Autodesk Inventor part; units mm, degrees
(part 4 of 4)
  spline S791 degree 2 poles (-83.876, -10.5733) (-84.1775, -10.5733) (-84.5737, -10.1697) (-84.5737, -9.8634) knots 0 0 0 1 2 2 2
  spline S792 degree 2 poles (-84.5737, -9.8634) (-84.5737, -9.613) (-84.372, -9.3018) (-84.1823, -9.2118) knots 0 0 0 1 2 2 2
  spline S793 degree 2 poles (-84.1823, -9.2118) (-83.9903, -9.1195) (-83.4579, -9.0465) (-83.1515, -9.0271) knots 0 0 0 1 2 2 2
  line L809 (-83.1515, -9.0271) -> (-83.1515, -9.0149)
  spline S794 degree 2 poles (-83.1515, -9.0149) (-83.1515, -8.8277) (-83.4287, -8.6843) (-83.7058, -8.6843) knots 0 0 0 1 2 2 2
  spline S795 degree 2 poles (-83.7058, -8.6843) (-83.8298, -8.6843) (-84.1653, -8.7742) (-84.3233, -8.8447) knots 0 0 0 1 2 2 2
  line L810 (-84.3233, -8.8447) -> (-84.3841, -8.8447)
  line L811 (-84.3841, -8.8447) -> (-84.3841, -8.2977)
  spline S796 degree 2 poles (-84.3841, -8.2977) (-84.2796, -8.2686) (-83.8128, -8.1859) (-83.5746, -8.1859) knots 0 0 0 1 2 2 2
  spline S797 degree 2 poles (-83.5746, -8.1859) (-82.9911, -8.1859) (-82.4562, -8.5749) (-82.4562, -8.9736) knots 0 0 0 1 2 2 2
  line L812 (-82.4562, -8.9736) -> (-82.4562, -10.5125)
  line L813 (-82.4562, -10.5125) -> (-83.1564, -10.5125)
  line L814 (-83.1564, -10.5125) -> (-83.1564, -10.2718)
  line L815 (-83.1564, -9.9217) -> (-83.1564, -9.4525)
  spline S798 degree 2 poles (-83.1564, -9.4525) (-83.3363, -9.4695) (-83.5575, -9.4963) (-83.6645, -9.5352) knots 0 0 0 1 2 2 2
  spline S799 degree 2 poles (-83.6645, -9.5352) (-83.7593, -9.5668) (-83.8614, -9.6981) (-83.8614, -9.805) knots 0 0 0 1 2 2 2
  spline S800 degree 2 poles (-83.8614, -9.805) (-83.8614, -9.9631) (-83.6888, -10.0822) (-83.5211, -10.0822) knots 0 0 0 1 2 2 2
  spline S801 degree 2 poles (-83.5211, -10.0822) (-83.4287, -10.0822) (-83.2342, -9.9971) (-83.1564, -9.9217) knots 0 0 0 1 2 2 2
  line L816 (-79.816, -10.5125) -> (-80.5259, -10.5125)
  line L817 (-80.5259, -10.5125) -> (-80.5259, -9.3917)
  spline S802 degree 2 poles (-80.5259, -9.3917) (-80.5259, -9.2532) (-80.5478, -8.9809) (-80.577, -8.9177) knots 0 0 0 1 2 2 2
  spline S803 degree 2 poles (-80.577, -8.9177) (-80.6135, -8.8399) (-80.7496, -8.7742) (-80.8663, -8.7742) knots 0 0 0 1 2 2 2
  spline S804 degree 2 poles (-80.8663, -8.7742) (-80.9514, -8.7742) (-81.1288, -8.8399) (-81.2285, -8.9104) knots 0 0 0 1 2 2 2
  line L818 (-81.2285, -8.9104) -> (-81.2285, -10.5125)
  line L819 (-81.2285, -10.5125) -> (-81.9335, -10.5125)
  line L820 (-81.9335, -10.5125) -> (-81.9335, -8.2491)
  line L821 (-81.9335, -8.2491) -> (-81.2285, -8.2491)
  line L822 (-81.2285, -8.2491) -> (-81.2285, -8.4995)
  spline S805 degree 2 poles (-81.2285, -8.4995) (-81.0559, -8.3537) (-80.7277, -8.1883) (-80.5284, -8.1883) knots 0 0 0 1 2 2 2
  spline S806 degree 2 poles (-80.5284, -8.1883) (-80.1831, -8.1883) (-79.816, -8.6259) (-79.816, -9.0392) knots 0 0 0 1 2 2 2
  line L823 (-79.816, -9.0392) -> (-79.816, -10.5125)
  line L824 (-78.5883, -10.5125) -> (-79.2934, -10.5125)
  line L825 (-79.2934, -10.5125) -> (-79.2934, -8.2491)
  line L826 (-79.2934, -8.2491) -> (-78.5883, -8.2491)
  line L827 (-78.5883, -8.2491) -> (-78.5883, -10.5125)
  line L828 (-78.5664, -7.9258) -> (-79.3128, -7.9258)
  line L829 (-79.3128, -7.9258) -> (-79.3128, -7.3763)
  line L830 (-79.3128, -7.3763) -> (-78.5664, -7.3763)
  line L831 (-78.5664, -7.3763) -> (-78.5664, -7.9258)
  spline S807 degree 2 poles (-76.94, -10.5733) (-77.2196, -10.5733) (-77.684, -10.4323) (-77.8566, -10.2864) knots 0 0 0 1 2 2 2
  spline S808 degree 2 poles (-77.8566, -10.2864) (-78.0243, -10.1381) (-78.2139, -9.6932) (-78.2139, -9.3917) knots 0 0 0 1 2 2 2
  spline S809 degree 2 poles (-78.2139, -9.3917) (-78.2139, -9.066) (-78.0097, -8.6114) (-77.8323, -8.4655) knots 0 0 0 1 2 2 2
  spline S810 degree 2 poles (-77.8323, -8.4655) (-77.6645, -8.3245) (-77.2075, -8.1883) (-76.9595, -8.1883) knots 0 0 0 1 2 2 2
  spline S811 degree 2 poles (-76.9595, -8.1883) (-76.7723, -8.1883) (-76.3979, -8.2759) (-76.2083, -8.3707) knots 0 0 0 1 2 2 2
  line L832 (-76.2083, -8.3707) -> (-76.2083, -8.9736)
  line L833 (-76.2083, -8.9736) -> (-76.2982, -8.9736)
  spline S812 degree 2 poles (-76.2982, -8.9736) (-76.342, -8.9323) (-76.4635, -8.835) (-76.5365, -8.7961) knots 0 0 0 1 2 2 2
  spline S813 degree 2 poles (-76.5365, -8.7961) (-76.6143, -8.7524) (-76.8063, -8.694) (-76.9254, -8.694) knots 0 0 0 1 2 2 2
  spline S814 degree 2 poles (-76.9254, -8.694) (-77.1953, -8.694) (-77.4919, -9.0708) (-77.4919, -9.3917) knots 0 0 0 1 2 2 2
  spline S815 degree 2 poles (-77.4919, -9.3917) (-77.4919, -9.7321) (-77.1759, -10.0676) (-76.9133, -10.0676) knots 0 0 0 1 2 2 2
  spline S816 degree 2 poles (-76.9133, -10.0676) (-76.7796, -10.0676) (-76.5802, -10.0068) (-76.5073, -9.9631) knots 0 0 0 1 2 2 2
  spline S817 degree 2 poles (-76.5073, -9.9631) (-76.4368, -9.9217) (-76.3347, -9.8293) (-76.2982, -9.7929) knots 0 0 0 1 2 2 2
  line L834 (-76.2982, -9.7929) -> (-76.2083, -9.7929)
  line L835 (-76.2083, -9.7929) -> (-76.2083, -10.3982)
  spline S818 degree 2 poles (-76.2083, -10.3982) (-76.269, -10.425) (-76.4271, -10.493) (-76.5097, -10.5149) knots 0 0 0 1 2 2 2
  spline S819 degree 2 poles (-76.5097, -10.5149) (-76.6118, -10.5441) (-76.7917, -10.5733) (-76.94, -10.5733) knots 0 0 0 1 2 2 2
  spline S820 degree 2 poles (-74.6256, -10.2718) (-74.6985, -10.3326) (-74.8128, -10.4298) (-74.91, -10.4785) knots 0 0 0 1 2 2 2
  spline S821 degree 2 poles (-74.91, -10.4785) (-75.0049, -10.5246) (-75.1848, -10.5733) (-75.3452, -10.5733) knots 0 0 0 1 2 2 2
  spline S822 degree 2 poles (-75.3452, -10.5733) (-75.6467, -10.5733) (-76.0429, -10.1697) (-76.0429, -9.8634) knots 0 0 0 1 2 2 2
  spline S823 degree 2 poles (-76.0429, -9.8634) (-76.0429, -9.613) (-75.8412, -9.3018) (-75.6515, -9.2118) knots 0 0 0 1 2 2 2
  spline S824 degree 2 poles (-75.6515, -9.2118) (-75.4595, -9.1195) (-74.9271, -9.0465) (-74.6207, -9.0271) knots 0 0 0 1 2 2 2
  line L836 (-74.6207, -9.0271) -> (-74.6207, -9.0149)
  spline S825 degree 2 poles (-74.6207, -9.0149) (-74.6207, -8.8277) (-74.8979, -8.6843) (-75.175, -8.6843) knots 0 0 0 1 2 2 2
  spline S826 degree 2 poles (-75.175, -8.6843) (-75.299, -8.6843) (-75.6345, -8.7742) (-75.7925, -8.8447) knots 0 0 0 1 2 2 2
  line L837 (-75.7925, -8.8447) -> (-75.8533, -8.8447)
  line L838 (-75.8533, -8.8447) -> (-75.8533, -8.2977)
  spline S827 degree 2 poles (-75.8533, -8.2977) (-75.7488, -8.2686) (-75.282, -8.1859) (-75.0438, -8.1859) knots 0 0 0 1 2 2 2
  spline S828 degree 2 poles (-75.0438, -8.1859) (-74.4603, -8.1859) (-73.9254, -8.5749) (-73.9254, -8.9736) knots 0 0 0 1 2 2 2
  line L839 (-73.9254, -8.9736) -> (-73.9254, -10.5125)
  line L840 (-73.9254, -10.5125) -> (-74.6256, -10.5125)
  line L841 (-74.6256, -10.5125) -> (-74.6256, -10.2718)
  line L842 (-74.6256, -9.9217) -> (-74.6256, -9.4525)
  spline S829 degree 2 poles (-74.6256, -9.4525) (-74.8055, -9.4695) (-75.0267, -9.4963) (-75.1337, -9.5352) knots 0 0 0 1 2 2 2
  spline S830 degree 2 poles (-75.1337, -9.5352) (-75.2285, -9.5668) (-75.3306, -9.6981) (-75.3306, -9.805) knots 0 0 0 1 2 2 2
  spline S831 degree 2 poles (-75.3306, -9.805) (-75.3306, -9.9631) (-75.158, -10.0822) (-74.9903, -10.0822) knots 0 0 0 1 2 2 2
  spline S832 degree 2 poles (-74.9903, -10.0822) (-74.8979, -10.0822) (-74.7034, -9.9971) (-74.6256, -9.9217) knots 0 0 0 1 2 2 2
  line L843 (-72.6977, -10.5125) -> (-73.4028, -10.5125)
  line L844 (-73.4028, -10.5125) -> (-73.4028, -7.3788)
  line L845 (-73.4028, -7.3788) -> (-72.6977, -7.3788)
  line L846 (-72.6977, -7.3788) -> (-72.6977, -10.5125)
  spline S833 degree 2 poles (-70.7796, -9.3601) (-70.7796, -9.664) (-70.8865, -10.2256) (-70.9814, -10.459) knots 0 0 0 1 2 2 2
  spline S834 degree 2 poles (-70.9814, -10.459) (-71.081, -10.707) (-71.3606, -11.1373) (-71.5308, -11.3415) knots 0 0 0 1 2 2 2
  line L847 (-71.5308, -11.3415) -> (-72.2699, -11.3415)
  line L848 (-72.2699, -11.3415) -> (-72.2699, -11.2832)
  spline S835 degree 2 poles (-72.2699, -11.2832) (-72.1094, -11.1397) (-71.8031, -10.7532) (-71.684, -10.5149) knots 0 0 0 1 2 2 2
  spline S836 degree 2 poles (-71.684, -10.5149) (-71.5575, -10.2645) (-71.4117, -9.7054) (-71.4117, -9.3601) knots 0 0 0 1 2 2 2
  spline S837 degree 2 poles (-71.4117, -9.3601) (-71.4117, -9.0295) (-71.5624, -8.446) (-71.684, -8.2054) knots 0 0 0 1 2 2 2
  spline S838 degree 2 poles (-71.684, -8.2054) (-71.8104, -7.9574) (-72.107, -7.583) (-72.2699, -7.4371) knots 0 0 0 1 2 2 2
  line L849 (-72.2699, -7.4371) -> (-72.2699, -7.3788)
  line L850 (-72.2699, -7.3788) -> (-71.5308, -7.3788)
  spline S839 degree 2 poles (-71.5308, -7.3788) (-71.3558, -7.5879) (-71.0762, -8.0206) (-70.9789, -8.2637) knots 0 0 0 1 2 2 2
  spline S840 degree 2 poles (-70.9789, -8.2637) (-70.8914, -8.4874) (-70.7796, -9.0271) (-70.7796, -9.3601) knots 0 0 0 1 2 2 2
  dimension "d12" = 95
  dimension "d14" = 45
  dimension "d15" = 27.5
  dimension "d16" = 2.5
  constraints: 4 other
  measures "d12" distance between parallel lines of L8 L10
  measures "d14" distance between parallel lines of L3 L1
  measures "d15" distance between parallel lines of L6 L1
  measures "d16" distance between parallel lines of L6 L8
extrude "Extrusion2" cut sketch "Sketch2" against normal blind 3 contours S0 S1 L12 L13 S2 S3 S4 L14 L15 L16 L17 L18 | S5 S6 S7 S8 L19 L20 S9 S10 S11 L21 L22 S12 S13 | L24 S18 S19 L25 L26 L27 L28 L29 S20 S21 L30 | L31 L32 L33 L34 | L35 L36 L37 L38 | S22 S23 S24 S25 S26 L39 L40 S27 S28 S29 S30 S31 L41 L42 S32 S33 | L43 L44 S34 S35 S36 L45 L46 L47 L48 L49 S37 S38 L50 | S39 S40 S41 S42 | S47 S48 S49 S50 S51 S52 L51 L52 S53 S54 S55 S56 S57 S58 S59 S60 L53 L54 S61 S62 | S63 S64 S65 S66 | L55 L56 S71 S72 S73 L57 L58 L59 S74 S75 S76 L60 L61 L62 | L63 L64 S77 S78 S79 L65 L66 L67 L68 L69 S80 S81 L70 | S82 L71 L72 S83 S84 S85 S86 S87 S88 S89 S90 S91 L73 L74 S92 S93 S94 S95 S96 S97 S98 | S99 S100 S101 S102 L75 L76 S103 S104 S105 L77 L78 S106 S107 | L80 L81 L82 L83 | S112 S113 S114 S115 S116 S117 S118 S119 | S126 L84 L85 L86 L87 L88 L89 L90 L91 L92 L93 L94 S127 S128 S129 L95 L96 S130 | L97 L98 L99 L100 | L101 L102 L103 L104 | S131 L105 L106 S132 S133 S134 S135 S136 S137 S138 S139 S140 L107 L108 S141 S142 S143 S144 S145 S146 S147 | S148 S149 S150 S151 S152 S153 L109 L110 S154 S155 S156 S157 S158 S159 L111 L112 L113 L114 L115 S160 S161 | L116 S162 S163 L117 L118 L119 L120 L121 S164 S165 L122 | S166 S167 S168 S169 S170 S171 L123 S172 S173 S174 L124 L125 S175 S176 S177 L126 L127 L128 | S182 S183 S184 S185 L130 L131 S186 S187 S188 L132 L133 S189 S190 | S195 L135 L136 L137 L138 L139 L140 L141 L142 L143 L144 L145 S196 S197 S198 L146 L147 S199 | L148 L149 L150 L151 L152 L153 L154 L155 L156 L157 | S200 S201 S202 S203 S204 S205 L158 L159 S206 S207 S208 S209 S210 S211 L160 L161 L162 L163 L164 S212 S213 | L165 L166 L167 L168 | S214 S215 S216 S217 L169 L170 S218 S219 S220 L171 L172 S221 S222 | L174 L175 S227 S228 S229 L176 L177 L178 L179 L180 S230 S231 L181 | L182 L183 S232 S233 S234 L184 L185 L186 L187 L188 S235 S236 L189 | L190 L191 L192 L193 L194 L195 | S237 S238 S239 S240 S241 S242 L196 S243 S244 S245 L197 L198 S246 S247 S248 L199 L200 L201 | L203 S253 S254 S255 S256 L204 L205 L206 S257 S258 S259 L207 L208 L209 L210 L211 S260 S261 S262 S263 S264 L212 L213 | S265 S266 L214 L215 L216 L217 L218 S267 S268 | S273 S274 S275 S276 L220 L221 S277 S278 S279 L222 L223 S280 S281 | L225 S286 S287 L226 L227 L228 L229 L230 S288 S289 L231 | S290 L232 L233 L234 L235 L236 L237 L238 L239 L240 L241 L242 S291 S292 S293 L243 L244 S294 | S295 S296 L245 L246 S297 S298 S299 L247 L248 L249 L250 L251 | S300 S301 S302 S303 | S308 S309 S310 S311 L252 L253 S312 S313 S314 L254 L255 S315 S316 | L257 L258 L259 L260 | S321 S322 L261 L262 L263 L264 L265 S323 S324 | L269 L270 L271 L272 | L273 L274 L275 L276 | S329 L277 L278 L279 L280 L281 L282 L283 L284 L285 L286 L287 S330 S331 S332 L288 L289 S333 | S334 S335 S336 S337 S338 S339 L290 S340 S341 S342 L291 L292 S343 S344 S345 L293 L294 L295 | S350 S351 L297 L298 S352 S353 S354 L299 L300 L301 L302 L303 | S355 S356 S357 S358 | S363 L304 L305 S364 S365 S366 S367 S368 S369 S370 S371 S372 L306 L307 S373 S374 S375 S376 S377 S378 S379 | L308 L309 S380 S381 S382 L310 L311 L312 L313 L314 S383 S384 L315 | L316 L317 S385 S386 S387 L318 L319 L320 S388 S389 S390 L321 L322 L323 | S391 S392 S393 S394 S395 S396 L324 S397 S398 S399 L325 L326 S400 S401 S402 L327 L328 L329 | L331 L332 L333 L334 L335 L336 L337 L338 L339 L340 L341 L342 | S407 S408 S409 S410 S411 S412 L343 S413 S414 S415 L344 L345 S416 S417 S418 L346 L347 L348 | S423 S424 L350 L351 L352 L353 L354 S425 S426 | L356 L357 S431 S432 S433 L358 L359 L360 S434 S435 S436 L361 L362 L363 | S437 L364 L365 S438 S439 S440 S441 S442 S443 S444 S445 S446 L366 L367 S447 S448 S449 S450 S451 S452 S453 | S454 S455 S456 S457 S458 S459 L368 S460 S461 S462 L369 L370 S463 S464 S465 L371 L372 L373 | L375 L376 S470 S471 S472 L377 L378 L379 L380 L381 S473 S474 L382 | S475 S476 S477 S478 S479 S480 L383 S481 S482 S483 L384 L385 S484 S485 S486 L386 L387 L388 | S491 L390 L391 S492 S493 S494 S495 S496 S497 S498 S499 L392 L393 S500 S501 S502 S503 S504 S505 S506 | L394 L395 L396 L397 | L398 L399 L400 L401 | L402 S507 S508 S509 S510 L403 L404 L405 S511 S512 S513 L406 L407 L408 L409 L410 S514 S515 S516 S517 S518 L411 L412 | L413 L414 L415 L416 L417 L418 L419 L420 L421 L422 L423 L424 L425 | L426 L427 L428 L429 | L430 L431 L432 L433 | L434 L435 S519 S520 S521 L436 L437 L438 L439 L440 S522 S523 L441 | S524 S525 L442 L443 S526 S527 S528 L444 L445 L446 L447 L448 | L449 L450 L451 L452 | L453 L454 L455 L456 | L457 L458 L459 L460 | S529 L461 L462 S530 S531 S532 S533 S534 S535 S536 S537 L463 L464 S538 S539 S540 S541 S542 S543 S544 | S545 S546 S547 S548 S549 S550 L465 S551 S552 S553 L466 L467 S554 S555 S556 L468 L469 L470 | L472 L473 L474 L475 L476 L477 L478 L479 | S561 S562 S563 S564 | L480 L481 L482 L483 L484 L485 L486 L487 L488 L489 L490 L491 L492 | S569 S570 S571 S572 S573 S574 L493 S575 S576 S577 L494 L495 S578 S579 S580 L496 L497 L498 | S585 S586 S587 L500 L501 S588 S589 S590 L502 L503 L504 L505 L506 | S591 S592 S593 L507 L508 S594 S595 S596 S597 S598 L509 L510 L511 S599 S600 S601 S602 S603 S604 L512 L513 S605 S606 S607 S608 L514 S609 S610 | S611 S612 S613 S614 S615 S616 L515 L516 S617 S618 S619 S620 S621 | S630 S631 S632 S633 S634 L517 S635 S636 S637 S638 S639 S640 L518 S641 | L519 L520 L521 L522 | L523 L524 L525 L526 | L527 L528 L529 L530 L531 L532 L533 L534 | S653 S654 L538 L539 L540 S655 S656 | L544 L545 L546 L547 L548 L549 L550 | L551 L552 L553 L554 L555 L556 L557 L558 | L562 L563 L564 L565 L566 L567 L568 L569 L570 L571 | S661 S662 S663 S664 L572 L573 S665 S666 S667 S668 S669 S670 S671 S672 L574 L575 S673 S674 | L576 L577 L578 L579 L580 L581 L582 L583 L584 L585 L586 L587 | S675 S676 L588 L589 L590 S677 S678 | S683 S684 L594 L595 L596 S685 S686 | L600 L601 L602 L603 L604 L605 L606 L607 L608 L609 L610 L611 | S691 S692 S693 L612 L613 L614 L615 L616 S694 S695 | L620 L621 L622 L623 L624 L625 | S701 S702 S703 S704 | L626 L627 L628 L629 L630 L631 L632 L633 L634 L635 L636 L637 L638 | L639 L640 L641 L642 L643 L644 L645 L646 | S713 S714 S715 S716 | L650 L651 L652 L653 L654 L655 L656 L657 L658 L659 | L660 L661 L662 L663 L664 L665 L666 L667 L668 L669 L670 L671 | L672 L673 L674 L675 L676 L677 L678 L679 L680 L681 | S725 S726 S727 S728 L682 L683 S729 S730 S731 S732 S733 S734 L684 L685 L686 L687 L688 | L689 L690 L691 L692 L693 L694 L695 L696 L697 L698 L699 L700 | L701 L702 L703 L704 L705 L706 L707 L708 L709 L710 | L711 L712 L713 L714 L715 L716 L717 L718 L719 L720 L721 L722 | L723 L724 L725 L726 L727 L728 L729 L730 L731 L732 L733 L734 | L735 L736 L737 L738 L739 L740 L741 S735 S736 S737 L742 | L746 L747 L748 L749 L750 L751 L752 L753 L754 L755 L756 L757 | L758 L759 L760 L761 L762 L763 L764 L765 L766 L767 | S742 S743 S744 S745 L768 L769 S746 S747 S748 S749 S750 S751 L770 L771 L772 L773 L774 | L775 S752 S753 S754 S755 L776 L777 S756 S757 S758 S759 L778 | L779 L780 L781 L782 L783 L784 L785 L786 L787 L788 L789 L790 L791 | S760 S761 S762 L792 L793 S763 S764 S765 S766 L794 L795 S767 S768 | S771 S772 S773 S774 S775 L797 L798 S776 S777 S778 S779 S780 S781 L799 L800 S782 S783 | L801 L802 S784 S785 S786 L803 L804 L805 L806 L807 S787 S788 L808 | S789 S790 S791 S792 S793 L809 S794 S795 L810 L811 S796 S797 L812 L813 L814 | L816 L817 S802 S803 S804 L818 L819 L820 L821 L822 S805 S806 L823 | L824 L825 L826 L827 | L828 L829 L830 L831 | S807 S808 S809 S810 S811 L832 L833 S812 S813 S814 S815 S816 S817 L834 L835 S818 S819 | S820 S821 S822 S823 S824 L836 S825 S826 L837 L838 S827 S828 L839 L840 L841 | L843 L844 L845 L846 | S833 S834 L847 L848 S835 S836 S837 S838 L849 L850 S839 S840
body "Solid1"
